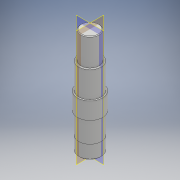
# Autodesk Inventor part: Вал тихоходный
Saved by Autodesk Inventor 2018.3 (Build 223284000, 284)
## iProperties
Created: 2018-03-24
Part Number: Вал тихоходный
Material: Типовые
Document SubType Name: Modeling
Designer: kriku
Density: 1 g/cm^3
Appearance: По умолчанию
Mass: 597.463 g
Surface Area: 497.082 cm^2
Volume: 597.463 cm^3
Author: kriku
Autodesk Inventor part; units mm, degrees
ref_plane "XY Plane" through (0, 0, 0) normal (0, 0, 1) x (1, 0, 0)
sketch "Эскиз1" plane through (0, 0, 0) normal (1, 0, 0) x (0, 1, 0)
  line L0 (22.5, 92.025) -> (22.5, 26.125)
  line L1 (22.5, 26.125) -> (27.5, 26.125)
  line L2 (27.5, 26.125) -> (27.5, -38.065)
  line L3 (27.5, -38.065) -> (28, -38.065)
  line L4 (28, -80.065) -> (28, -133.065)
  line L5 (28, -133.065) -> (27.5, -133.065)
  line L6 (27.5, -133.065) -> (27.5, -165.065)
  line L7 (25.5, -167.065) -> (0, -167.065)
  line L8 (0, -167.065) -> (0, 93.625)
  line L9 (0, 93.625) -> (20.9, 93.625)
  line L10 (27.5, -165.065) -> (25.5, -167.065)
  line L11 (28, -38.065) -> (31, -38.065)
  line L12 (31, -38.065) -> (31, -80.065)
  line L13 (31, -80.065) -> (28, -80.065)
  line L14 (20.9, 93.625) -> (22.5, 92.025)
  point P0 (0, 0)
  point P1 (27.5, -167.065)
  point P2 (22.5, 93.625)
  dimension "d0" = 45
  dimension "d1" = 55
  dimension "d2" = 56
  dimension "d3" = 67.5
  dimension "d7" = 34
  dimension "d8" = 2
  dimension "d9" = 2
  dimension "d11" = 62
  dimension "d13" = 42
  dimension "d14" = 53
  dimension "d15" = 1.6
  dimension "d16" = 1.6
  constraints: 30 end point, 10 perpendicular, 6 point on line, 1 horizontal, 1 vertical
  measures "d0" diameter of L0 L8
  measures "d1" diameter of L2 L8
  measures "d2" diameter of L4 L8
  measures "d3" distance of point (22.5, 93.625) L0.end
  measures "d7" distance of L5.end point (27.5, -167.065)
  measures "d8" distance of L6.end point (27.5, -167.065)
  measures "d9" distance of L7.start point (27.5, -167.065)
  measures "d11" diameter of L12 L8
  measures "d13" distance of L11.end L12.end
  measures "d14" distance of L4.start L4.end
  measures "d15" distance of L9.end point (22.5, 93.625)
  measures "d16" distance of L0.start point (22.5, 93.625)
revolve "Вращение1" add sketch "Эскиз1" angle 360 about axis through (0, 0, -167.065) along (0, 0, 1)
equation "\"d9\" = d8"
equation "\"d16\" = d15"
